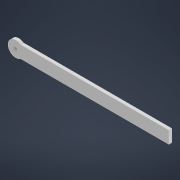
# Autodesk Inventor part: Рычаг_2
Saved by Autodesk Inventor 2021.2 (Build 252289000, 289)
## iProperties
Created: 2021-05-30
Part Number: Рычаг_2
Material: Типовые
Document SubType Name: Modeling
Designer: Admin
Density: 1 g/cm^3
Appearance: По умолчанию
Author: Admin
Autodesk Inventor part; units mm, degrees
ref_plane "YZ Plane" through (0, 0, 0) normal (1, 0, 0) x (0, 1, 0)
ref_plane "XZ Plane" through (0, 0, 0) normal (0, 1, 0) x (-1, 0, 0)
ref_plane "XY Plane" through (0, 0, 0) normal (0, 0, 1) x (1, 0, 0)
sketch "Эскиз1" plane through (0, 0, 0) normal (0, 0, 1) x (1, 0, 0)
  arc A0 (30, 40) -> (30, -40) centre (0, 0) ccw
  line L0 (30, 40) -> (1000, 40)
  line L1 (1000, 40) -> (1000, -40)
  line L2 (1000, -40) -> (30, -40)
  dimension "d0" = 100
  dimension "d1" = 1000
  dimension "d4" = 80
  dimension "d5" = 40
  constraints: 6 end point, 2 horizontal, 2 point on circle, 1 centre point, 1 coincident, 1 vertical
  measures "d0" diameter of A0
  measures "d1" distance from line of L1 point (0, 0)
  measures "d4" distance between parallel lines of L2 L0
  measures "d5" distance from line of L0 point (0, 0)
extrude "Выдавливание1" add sketch "Эскиз1" along normal blind 20
sketch "Эскиз2" plane through (0, 0, 20) normal (0, 0, 1) x (1, 0, 0)
  point P0 (0, 0)
  point P1 (0, 0)
  constraints: 1 coincident
hole "Отверстие1" at (0, 0, 20) direction (0, 0, -1) diameter 18 end through all
